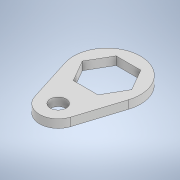
# Autodesk Inventor part: palanca2
Saved by Autodesk Inventor 2021.2 (Build 252289000, 289)
## iProperties
Created: 2026-06-16
Part Number: palanca2
Material: Generic
Document SubType Name: Sheet Metal
Designer: nelso
Density: 1 g/cm^3
Sheet Metal Rule: Default_mm
Appearance: Default
Author: nelso
Autodesk Inventor part; units mm, degrees
ref_plane "YZ Plane" through (0, 0, 0) normal (1, 0, 0) x (0, 1, 0)
ref_plane "XZ Plane" through (0, 0, 0) normal (0, 1, 0) x (-1, 0, 0)
ref_plane "XY Plane" through (0, 0, 0) normal (0, 0, 1) x (1, 0, 0)
sketch "Sketch1" plane through (0, 0, 0) normal (0, 1, 0) x (-1, 0, 0)
  circle A0 centre (0, 0) radius 3
  circle A1 centre (0, 0) radius 7
  circle A2 centre (0, -18.2266) radius 12.5
  line L0 (6.6737, 2.1123) -> (11.9173, -14.4547)
  line L1 (-11.9173, -14.4547) -> (-6.6737, 2.1123)
  line L2 (9.2376, -18.2266) -> (4.6188, -26.2266)
  line L3 (4.6188, -26.2266) -> (-4.6188, -26.2266)
  line L4 (-4.6188, -26.2266) -> (-9.2376, -18.2266)
  line L5 (-9.2376, -18.2266) -> (-4.6188, -10.2266)
  line L6 (-4.6188, -10.2266) -> (4.6188, -10.2266)
  line L7 (4.6188, -10.2266) -> (9.2376, -18.2266)
  point P0 (4.4139, 5.433)
  point P1 (-8.9361, -9.4862)
  dimension "d3" = 6
  dimension "d6" = 14
  dimension "d11" = 18.2266
  dimension "d12" = 25
  dimension "d13" = 16
  measures "d3" diameter of A0
  measures "d6" diameter of A1
  measures "d11" distance of A2.centre A0.centre
  measures "d12" diameter of A2
  measures "d13" distance between parallel lines of L3 L6
extrude "Plate1" add sketch "Sketch1" along normal mid plane 3.1
equation "\"d9\" = Thickness"
equation "\"BendRadius\" = Thickness"
equation "\"BendReliefWidth\" = Thickness"
equation "\"BendReliefDepth\" = 0.5 * Thickness"
equation "\"CornerReliefSize\" = 4 * Thickness"
equation "\"MinimumRemnant\" = 2 * Thickness"
equation "\"TransitionRadius\" = BendRadius"
equation "\"JacobiRadiusSize\" = BendRadius"
equation "\"GapSize\" = Thickness"
equation "\"Thickness\" = 3.1"
body "Solid1"
